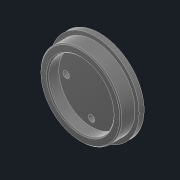
# Autodesk Inventor part: base13
Saved by Autodesk Inventor 2022 (Build 260153000, 153)
## iProperties
Created: 2021-07-12
Part Number: base13
Material: ABS プラスチック
Document SubType Name: Modeling
Designer: yuta0
Density: 1.06 g/cm^3
Appearance: 滑らか - 黒
購入先: 印刷
在庫数: 0.0
Author: yuta0
Autodesk Inventor part; units mm, degrees
ref_plane "YZ Plane" through (0, 0, 0) normal (1, 0, 0) x (0, 1, 0)
ref_plane "XZ Plane" through (0, 0, 0) normal (0, 1, 0) x (-1, 0, 0)
ref_plane "XY Plane" through (0, 0, 0) normal (0, 0, 1) x (1, 0, 0)
sketch "スケッチ1" plane through (0, 0, 0) normal (1, 0, 0) x (0, 1, 0)
  line L0 (21.95, 0) -> (21.95, 2.5)
  line L1 (21.95, 2.5) -> (19.95, 2.5)
  line L2 (19.95, 2.5) -> (19.95, 9.5)
  line L3 (19.95, 9.5) -> (0, 9.5)
  line L4 (0, 9.5) -> (0, 0)
  line L5 (0, 0) -> (21.95, 0)
  dimension "d0" = 19.95
  dimension "d1" = 7
  dimension "d2" = 2.5
  dimension "d3" = 2
  constraints: 12 end point, 5 perpendicular, 1 vertical
  measures "d0" distance of L2.end L3.end
  measures "d1" distance of L1.end L2.end
  measures "d2" distance of L0.start L0.end
  measures "d3" distance of L0.end L1.end
revolve "回転1" add sketch "スケッチ1" angle 360 about axis through (0, 0, 9.5) along (0, 0, -1)
chamfer "面取り1" distance 0.5 angle 45 1 edges at (0, -19.95, 9.5)
sketch "スケッチ4" plane through (0, 0, 9.5) normal (0, 0, 1) x (1, 0, 0)
  circle A0 centre (0, 0) radius 12.5
  point P0 (0, 0)
  point P1 (0, 12.5)
  point P2 (-12.5, 0)
  point P3 (0, -12.5)
  point P4 (12.5, 0)
  dimension "d13" = 25
  dimension "d16" = 360
  constraints: 1 coincident, 1 vertical alignment, 7 other
hole "穴1" at (0, 12.5, 9.5) at (-12.5, 0, 9.5) at (0, -12.5, 9.5) at (12.5, 0, 9.5) direction (0, 0, -1) diameter 3.2 end through all clearance for "Flat Head Machine Screw" size "M3" standard "Ansi Metric M Profile"
sketch "スケッチ5" plane through (0, 0, 9.5) normal (0, 0, 1) x (1, 0, 0)
  circle A0 centre (0, 0) radius 16.15
  point P0 (0, 0)
  dimension "d30" = 32.3
  constraints: 1 centre point, 1 coincident
  measures "d30" diameter of A0
extrude "押し出し4" cut sketch "スケッチ5" against normal blind 5.5
chamfer "面取り2" distance 0.5 angle 45 1 edges at (-16.15, 0, 9.5)
